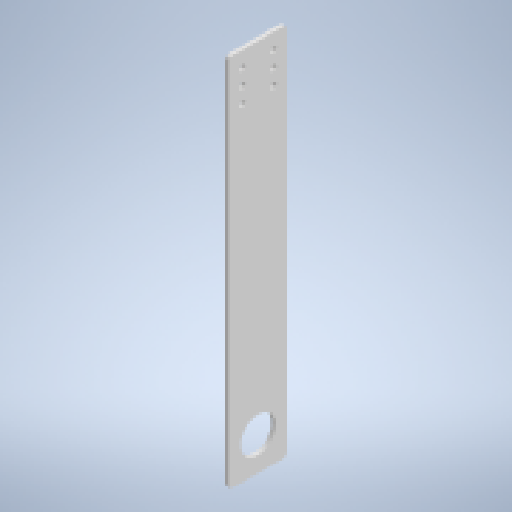
# Autodesk Inventor part: Drop for pivot intake
Saved by Autodesk Inventor 2023 (Build 270158000, 158)
## iProperties
Created: 2023-03-19
Part Number: Drop for pivot intake
Material: Generic
Document SubType Name: Modeling
Designer: Gabriel - T3 CAD
Density: 1 g/cm^3
Appearance: Default
Author: Gabriel - T3 CAD
Autodesk Inventor part; units mm, degrees
ref_plane "YZ Plane" through (0, 0, 0) normal (1, 0, 0) x (0, 1, 0)
ref_plane "XZ Plane" through (0, 0, 0) normal (0, 1, 0) x (-1, 0, 0)
ref_plane "XY Plane" through (0, 0, 0) normal (0, 0, 1) x (1, 0, 0)
sketch "Sketch1" plane through (0, 0, 0) normal (1, 0, 0) x (0, 1, 0)
  line L0 (-3.175, 0) -> (-301.625, 0)
  line L1 (-304.8, 3.175) -> (-304.8, 44.45)
  line L2 (-301.625, 47.625) -> (-3.175, 47.625)
  line L3 (0, 44.45) -> (0, 3.175)
  circle A0 centre (-277.8125, 23.8125) radius 14.2875
  arc A1 (0, 44.45) -> (-3.175, 47.625) centre (-3.175, 44.45) ccw
  arc A2 (-3.175, 0) -> (0, 3.175) centre (-3.175, 3.175) ccw
  arc A3 (-304.8, 3.175) -> (-301.625, 0) centre (-301.625, 3.175) ccw
  arc A4 (-301.625, 47.625) -> (-304.8, 44.45) centre (-301.625, 44.45) ccw
  circle A5 centre (-12.7, 36.5125) radius 2.3813
  circle A6 centre (-25.4, 36.5125) radius 2.3813
  circle A7 centre (-38.1, 36.5125) radius 2.3813
  circle A8 centre (-12.7, 11.1125) radius 2.3813
  circle A9 centre (-25.4, 11.1125) radius 2.3813
  circle A10 centre (-38.1, 11.1125) radius 2.3813
  circle A11 centre (-50.8, 36.5125) radius 2.3813
  circle A12 centre (-50.8, 11.1125) radius 2.3813
  circle A13 centre (-63.5, 36.5125) radius 2.3813
  circle A14 centre (-63.5, 11.1125) radius 2.3813
  circle A15 centre (-76.2, 36.5125) radius 2.3813
  circle A16 centre (-76.2, 11.1125) radius 2.3813
  circle A17 centre (-88.9, 36.5125) radius 2.3813
  circle A18 centre (-88.9, 11.1125) radius 2.3813
  circle A19 centre (-101.6, 36.5125) radius 2.3813
  circle A20 centre (-101.6, 11.1125) radius 2.3813
  circle A21 centre (-114.3, 36.5125) radius 2.3813
  circle A22 centre (-114.3, 11.1125) radius 2.3813
  circle A23 centre (-127, 36.5125) radius 2.3813
  circle A24 centre (-127, 11.1125) radius 2.3813
  circle A25 centre (-139.7, 36.5125) radius 2.3813
  circle A26 centre (-139.7, 11.1125) radius 2.3813
  circle A27 centre (-152.4, 36.5125) radius 2.3813
  circle A28 centre (-152.4, 11.1125) radius 2.3813
  circle A29 centre (-165.1, 36.5125) radius 2.3813
  circle A30 centre (-165.1, 11.1125) radius 2.3813
  circle A31 centre (-177.8, 36.5125) radius 2.3813
  circle A32 centre (-177.8, 11.1125) radius 2.3813
  circle A33 centre (-190.5, 36.5125) radius 2.3813
  circle A34 centre (-190.5, 11.1125) radius 2.3813
  circle A35 centre (-203.2, 36.5125) radius 2.3813
  circle A36 centre (-203.2, 11.1125) radius 2.3813
  circle A37 centre (-215.9, 36.5125) radius 2.3813
  circle A38 centre (-215.9, 11.1125) radius 2.3813
  point P0 (0, 0)
  point P1 (-304.8, 47.625)
  point P2 (-304.8, 0)
  point P3 (0, 47.625)
  dimension "d0" = 304.8
  dimension "d1" = 47.625
  dimension "d4" = 26.9875
  dimension "d5" = 28.575
  dimension "d6" = 3.175
  dimension "d9" = 23.8125
  dimension "d18" = 11.1125
  dimension "d19" = 4.7625
  dimension "d20" = 12.7
  dimension "d23" = 12.7
  dimension "d26" = 25.4
  constraints: 39 centre point, 8 end point, 8 point on circle, 8 point on line, 8 tangent, 3 equal radius, 2 horizontal, 2 parallel, 1 perpendicular, 1 vertical, 66 other
  measures "d0" distance of point (-304.8, 47.625) point (0, 47.625)
  measures "d1" distance of point (-304.8, 0) point (-304.8, 47.625)
  measures "d4" distance from line of L1 A0.centre
  measures "d5" diameter of A0
  measures "d6" radius of A1
  measures "d9" distance from line of L0 A0.centre
  measures "d18" distance from line of L2 A5.centre
  measures "d19" diameter of A5
  measures "d20" distance from line of L3 A5.centre
  measures "d23" distance of A5.centre A6.centre
  measures "d26" distance of A5.centre A8.centre
extrude "Extrusion1" add sketch "Sketch1" along normal blind 3.175
equation "\"d9\" = 0.5 * d1"
equation "\"d18\" = -0.5 * d15 + 0.5 * d1"
equation "\"d15\" = 25.4"
body "Solid1"
